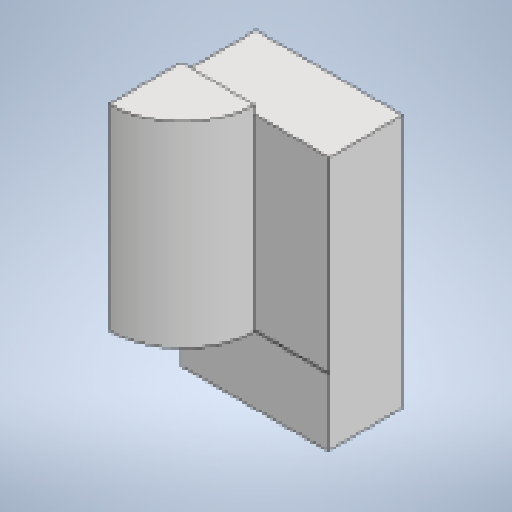
# Autodesk Inventor part: BSH 01 bag
Saved by Autodesk Inventor 2025.1 (Build 291241020, 241B)
## iProperties
Created: 2024-08-27
Part Number: BSH 01 bag
Material: Generic
Document SubType Name: Modeling
Designer: DELL
Density: 1 g/cm^3
Appearance: Default
Author: DELL
Autodesk Inventor part; units mm, degrees
ref_plane "YZ Plane" through (0, 0, 0) normal (1, 0, 0) x (0, 1, 0)
ref_plane "XZ Plane" through (0, 0, 0) normal (0, 1, 0) x (-1, 0, 0)
ref_plane "XY Plane" through (0, 0, 0) normal (0, 0, 1) x (1, 0, 0)
sketch "Sketch1" plane through (0, 0, 0) normal (0, 0, 1) x (1, 0, 0)
  line L0 (550, 275) -> (-550, 275)
  line L1 (-550, 275) -> (-550, -275)
  line L2 (-550, -275) -> (550, -275)
  line L3 (550, -275) -> (550, 275)
  line L4 (550, 275) -> (-550, -275) construction
  line L5 (-550, 275) -> (550, -275) construction
  point P0 (0, 0)
  dimension "d0" = 1100
  dimension "d1" = 550
  constraints: 12 end point, 2 midpoint, 2 parallel, 1 horizontal, 1 perpendicular
  measures "d0" distance of L2.end L1.end
  measures "d1" distance of L1.end L0.end
extrude "Extrusion1" add sketch "Sketch1" along normal blind 1900
sketch "Sketch2" plane through (-550, -275, 0) normal (0, -1, 0) x (1, 0, 0)
  line L0 (0, 0) -> (1100, 0) projected
  line L1 (1100, 0) -> (1100, 1900) projected
  line L2 (0, 1900) -> (1100, 1900) projected
  line L3 (0, 0) -> (0, 1900) projected
  line L4 (0, 500) -> (1100, 500)
  line L5 (845.0983, 500) -> (550, 1900)
  point P0 (550, 0)
  dimension "d4" = 500
  constraints: 4 end point, 3 point on line, 1 midpoint, 1 perpendicular
  measures "d4" distance between parallel lines of L0 L4
extrude "Extrusion2" add sketch "Sketch2" along normal blind 10 contours L3 L4 L1 L0
sketch "Sketch3" plane through (-550, -275, 500) normal (0, 0, 1) x (1, 0, 0)
  line L0 (0, 0) -> (1100, 0) projected
  line L1 (0, 0) -> (0, -10) projected
  line L2 (1100, -10) -> (0, -10) projected
  line L3 (1100, 0) -> (1100, -10) projected
  circle A0 centre (0, 0) radius 550.0909
  line L4 (0, 0) -> (0, -550.0909)
  point P0 (550, 275)
  point P1 (550, -10)
  constraints: 2 end point, 2 point on circle, 1 centre point, 1 coincident, 1 midpoint, 1 vertical
extrude "Extrusion3" add sketch "Sketch3" along normal blind 1169 contours L2 A0 L4
body "Solid1"
